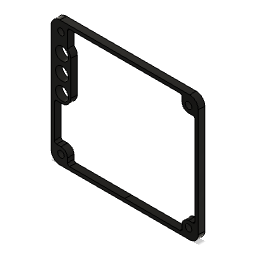
Logger gasket v17 (Autodesk Fusion 360 design; units mm, degrees)
Autodesk Fusion 360 part; units mm, degrees
sketch "Sketch1" plane through (0, 0, 0) normal (0, 0, 1) x (1, 0, 0)
  line L0 (-29.5, 24.5) -> (-35.5, 24.5) construction
  circle A0 centre (29.5, 24.5) radius 1.5
  line L1 (25.5009, -27.5) -> (3.5, -27.5)
  arc A1 (34, 25) -> (30, 29) centre (30, 25) ccw
  circle A2 centre (29.5, -24.5) radius 1.5
  arc A3 (30, -29) -> (34, -25) centre (30, -25) ccw
  line L2 (30, -29) -> (-30, -29)
  arc A4 (-34, -25) -> (-30, -29) centre (-30, -25) ccw
  line L3 (0, -27.5) -> (0.5, -27.5) construction
  line L4 (0.5, -27.5) -> (-25.5, -27.5)
  line L5 (-30, 29) -> (30, 29)
  line L6 (0, 27.5) -> (0.5, 27.5) construction
  circle A5 centre (-29.5, 24.5) radius 1.5
  arc A6 (-30, 29) -> (-34, 25) centre (-30, 25) ccw
  line L7 (0, -27.5) -> (0.5, -27.5) construction
  line L8 (-34, -25) -> (-34, 25)
  circle A7 centre (-29.5, -24.5) radius 1.5
  line L9 (0, -27.5) -> (0.5, -27.5)
  line L10 (34, 25) -> (34, -25)
  line L11 (-29.5, 24.5) -> (-34, 24.5) construction
  line L12 (-34, 24.5) -> (-34, 29) construction
  line L13 (-34, 29) -> (-29.5, 29) construction
  line L14 (-29.5, 29) -> (-29.5, 24.5) construction
  line L15 (-34, 29) -> (-29, 29) construction
  line L16 (-29, 29) -> (-29, 16) construction
  line L17 (-29, 16) -> (-34, 16) construction
  line L18 (-34, 16) -> (-34, 29) construction
  line L19 (-25, 13) -> (-25, 11)
  line L20 (-25, 5) -> (-25, 3)
  line L21 (-25, 13) -> (-25, 16)
  line L22 (-25, 11) -> (-25, 5)
  line L23 (-25, 3) -> (-25, 0)
  line L24 (-26.5, 24.4915) -> (-26.494, 26.6091)
  line L25 (-26.5, 24.4915) -> (-26.5151, 19.1346)
  arc A8 (-25.5, 27.5) -> (-26.4946, 26.3966) centre (-25.5, 26.5) ccw
  line L26 (-30, 27.5) -> (-29, 27.5)
  line L27 (-25.5, 27.5) -> (0.5, 27.5)
  arc A9 (-29, 27.458) -> (-29.5, 27.5) centre (-29.5, 24.5) ccw
  arc A10 (-29, 27.458) -> (-29.5, 27.5) centre (-29.5, 24.5) ccw
  circle A11 centre (-29, 16) radius 3
  circle A12 centre (-29, 8) radius 3
  circle A13 centre (-29, 0) radius 3
  arc A14 (-25, 16) -> (-26.5151, 19.1346) centre (-29, 16) ccw
  arc A15 (-29, -4) -> (-25, 0) centre (-29, 0) ccw
  line L28 (-32.5, -20.5009) -> (-32.5, -4.999)
  line L29 (-29, -3) -> (-29, -4) construction
  line L30 (-29, -4) -> (-31.5, -4)
  line L31 (-29.5, -24.5) -> (-26.5, -24.5) construction
  line L32 (-26.5, -24.5) -> (-26.5, -21.5) construction
  line L33 (-26.5, -21.5) -> (-29.5, -21.5) construction
  line L34 (-29.5, -21.5) -> (-29.5, -24.5) construction
  line L35 (-26.5, -24.5) -> (-26.5, -26.5)
  line L36 (-29.5, -21.5) -> (-31.5, -21.5)
  arc A16 (-26.5, -24.5015) -> (-29.5014, -21.5) centre (-29.5, -24.5) ccw
  arc A17 (-31.5, -4) -> (-32.5, -5.001) centre (-31.5, -5) ccw
  arc A18 (-32.5, -20.4991) -> (-31.5, -21.5) centre (-31.5, -20.5) ccw
  arc A19 (-26.5, -26.5) -> (-25.5, -27.5) centre (-25.5, -26.5) ccw
  line L37 (0.5, 27.5) -> (3.5, 27.5)
  line L38 (3.5, -27.5) -> (0.5, -27.5)
  line L39 (29.5, -24.5) -> (26.5, -24.5) construction
  line L40 (26.5, -24.5) -> (26.5, -21.5) construction
  line L41 (26.5, -21.5) -> (29.5, -21.5) construction
  line L42 (29.5, -21.5) -> (29.5, -24.5) construction
  line L43 (29.5, -21.5) -> (31.5, -21.5)
  line L44 (26.5, -24.5) -> (26.5, -26.5)
  line L45 (32.5, -24.5) -> (32.5, -25)
  arc A20 (29.5014, -21.5) -> (26.5, -24.5015) centre (29.5, -24.5) ccw
  arc A21 (25.4991, -27.5) -> (26.5, -26.5) centre (25.5, -26.5) ccw
  arc A22 (31.5, -21.5) -> (32.5, -20.5) centre (31.5, -20.5) ccw
  line L46 (29.5, 24.5) -> (26.5, 24.5) construction
  line L47 (26.5, 24.5) -> (26.5, 21.5) construction
  line L48 (26.5, 21.5) -> (29.5, 21.5) construction
  line L49 (29.5, 21.5) -> (29.5, 24.5) construction
  line L50 (26.5, 24.5) -> (26.5, 26.5)
  line L51 (29.5, 21.5) -> (31.5, 21.5)
  line L52 (32.5, 25) -> (32.5, 24.5)
  line L53 (32.5, 20.501) -> (32.5, -20.5)
  arc A23 (26.5, 24.5015) -> (29.5014, 21.5) centre (29.5, 24.5) ccw
  line L54 (3.5, 27.5) -> (25.5, 27.5)
  line L55 (29.5, 27.5) -> (30, 27.5)
  arc A24 (26.5, 26.5) -> (25.5, 27.5) centre (25.5, 26.5) ccw
  arc A25 (32.5, 20.499) -> (31.5, 21.5) centre (31.5, 20.5) ccw
  point P0 (-29, 12)
  dimension "d1" = 3
  dimension "d2" = 3
  dimension "d3" = 3
  dimension "d4" = 3
  dimension "d12" = 5
  dimension "d13" = 13
  dimension "d20" = 2
  constraint horizontal L2
  constraint perpendicular L2 L8
  constraint parallel L2 L5
  constraint parallel L8 L10
  constraint tangent L5 A6
  constraint tangent A6 L8
  constraint horizontal L1
  constraint perpendicular L1 L28
  constraint parallel L1 L26
  constraint parallel L28 L52
  constraint coincident L3.end L1
  constraint parallel L6 L26
  constraint collinear L1 L4
  constraint coincident L3.start L1
  constraint collinear L26 L54
  constraint coincident L6.start L26
  constraint horizontal L11
  constraint vertical L12
  constraint horizontal L13
  constraint vertical L14
  constraint horizontal L15
  constraint vertical L16
  constraint horizontal L17
  constraint vertical L18
  constraint tangent L23 A15
  constraint tangent A8 L26
  constraint coincident L24 A8.end
  constraint coincident A8.start L26
  constraint collinear L26 L27
  constraint coincident A8 L24.end
  constraint coincident L16 L26.end
  constraint coincident L14 A9.end
  constraint coincident L16 A9.start
  constraint concentric A13 A15
  constraint parallel L28 L29
  constraint tangent A15 L30
  constraint coincident A13 L29.start
  constraint concentric A7 A16
  constraint tangent L4 A16
  constraint horizontal L31
  constraint vertical L32
  constraint horizontal L33
  constraint vertical L34
  constraint coincident A7.centre L31.start
  constraint perpendicular L4 L35
  constraint perpendicular L28 L36
  constraint coincident L36 A16.end
  constraint coincident L35 A16.start
  constraint tangent L30 A17
  constraint coincident L28.end A17
  constraint coincident L28 A17.end
  constraint tangent L36 A18
  constraint coincident L28 A18.start
  constraint coincident A18 L28.start
  constraint tangent L4 A19
  constraint parallel L37 L54
  constraint concentric A2 A20
  constraint tangent L1 A20
  constraint horizontal L39
  constraint vertical L40
  constraint horizontal L41
  constraint vertical L42
  constraint coincident A2.centre L39.start
  constraint perpendicular L43 L52
  constraint perpendicular L1 L44
  constraint collinear L45 L52
  constraint coincident L43 A20.start
  constraint coincident L44 A20.end
  constraint tangent A22 L52
  constraint tangent L44 A21
  constraint coincident L1.start A21
  constraint coincident L1 A21.start
  constraint concentric A0 A23
  constraint tangent A23 L54
  constraint horizontal L46
  constraint vertical L47
  constraint horizontal L48
  constraint vertical L49
  constraint coincident A0.centre L46.start
  constraint perpendicular L50 L54
  constraint perpendicular L51 L52
  constraint collinear L52 L53
  constraint coincident L51 A23.end
  constraint coincident L55.start L54
  constraint collinear L54 L55
  constraint coincident L50 A23.start
  constraint tangent L51 A25
  constraint tangent L54 A24
  constraint coincident L53 A25.start
  constraint coincident A25 L53.start
  measures "d1" diameter of A5
  measures "d2" diameter of A0
  measures "d3" diameter of A2
  measures "d4" diameter of A7
  measures "d12" distance of L12.end L15.end
  measures "d13" distance of L12.end L17.end
  measures "d20" distance of L20.start L20.end
extrude "Extrude1" add sketch "Sketch1" along normal blind 3
equation "gasket_thikness = 3 mm"
equation "d21 = gasket_thikness"
